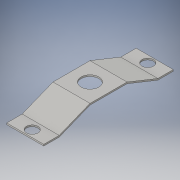
# Autodesk Inventor part: Up_cam_support
Saved by Autodesk Inventor 2016 (Build 200138000, 138)
## iProperties
Created: 2015-09-28
Part Number: Up_cam_support
Material: Generic
Document SubType Name: Modeling
Designer: fei
Density: 1 g/cm^3
Appearance: Default
Author: fei
Autodesk Inventor part; units mm, degrees
ref_plane "YZ Plane" through (0, 0, 0) normal (1, 0, 0) x (0, 1, 0)
ref_plane "XZ Plane" through (0, 0, 0) normal (0, 1, 0) x (-1, 0, 0)
ref_plane "XY Plane" through (0, 0, 0) normal (0, 0, 1) x (1, 0, 0)
sketch "Sketch1" plane through (0, 0, 0) normal (1, 0, 0) x (0, 1, 0)
  line L0 (174.9139, 1066.8) -> (200.3139, 1066.8)
  line L1 (200.3139, 1066.8) -> (200.3139, 812.8)
  line L2 (200.3139, 812.8) -> (403.5139, 304.8)
  line L3 (403.5139, 304.8) -> (403.5139, -304.8)
  line L4 (403.5139, -304.8) -> (200.3139, -812.8)
  line L5 (200.3139, -812.8) -> (200.3139, -1066.8)
  line L6 (174.9139, 1066.8) -> (174.9139, 812.8)
  line L7 (174.9139, 812.8) -> (378.1139, 304.8)
  line L8 (378.1139, 304.8) -> (378.1139, -304.8)
  line L9 (174.9139, -935.25) -> (174.9139, 993.0491) construction
  line L10 (174.9139, 681.698) -> (174.9139, -514.0179) construction
  line L11 (200.3139, -1066.8) -> (174.9139, -1066.8)
  line L12 (378.1139, -304.8) -> (174.9139, -812.8)
  line L13 (174.9139, -812.8) -> (174.9139, -1066.8)
  point P0 (0, 0)
  dimension "d0" = 254
  dimension "d1" = 508
  dimension "d2" = 609.6
  dimension "d3" = 508
  dimension "d4" = 254
  dimension "d6" = 304.8
  dimension "d8" = 25.4
  dimension "d10" = 203.2
  dimension "d26" = 25.4
  constraints: 28 end point, 6 point on line, 4 horizontal alignment, 3 vertical, 2 horizontal, 2 parallel, 1 collinear, 1 perpendicular
  measures "d0" distance of L0.end L1.end
  measures "d1" vertical distance of L1.end L2.end
  measures "d2" distance of L2.end L3.end
  measures "d3" vertical distance of L3.end L4.end
  measures "d4" distance of L4.end L5.end
  measures "d6" vertical distance of L2.end point (0, 0)
  measures "d8" distance of L0.start L0.end
  measures "d10" distance between parallel lines of L8 L9
  measures "d26" distance between parallel lines of L8 L3
extrude "Extrusion1" add sketch "Sketch1" along normal mid plane 609.6
sketch "Sketch2" plane through (-304.8, 200.3139, -812.8) normal (0, 1, 0) x (1, 0, 0)
  circle A0 centre (304.8, 139.7) radius 95.25
  line L0 (609.6, 254) -> (0, 254) projected
  line L1 (0, 0) -> (0, 254) projected
  circle A1 centre (304.8, -1765.3) radius 95.25
  line L2 (609.6, -1879.6) -> (0, -1879.6) projected
  line L3 (609.6, -1625.6) -> (609.6, -1879.6) projected
  point P0 (304.8, -812.8)
  dimension "d13" = 190.5
  dimension "d14" = 114.3
  dimension "d15" = 304.8
  dimension "d16" = 190.5
  dimension "d17" = 114.3
  dimension "d18" = 304.8
  constraints: 2 centre point
  measures "d13" diameter of A0
  measures "d14" distance from line of L0 A0.centre
  measures "d15" distance from line of L1 A0.centre
  measures "d16" diameter of A1
  measures "d17" distance from line of L2 A1.centre
  measures "d18" distance from line of L3 A1.centre
extrude "Extrusion2" cut sketch "Sketch2" against normal up to next
sketch "Sketch3" plane through (-304.8, 403.5139, 304.8) normal (0, 1, 0) x (1, 0, 0)
  circle A0 centre (304.8, 304.8) radius 146.05
  line L0 (0, 609.6) -> (0, 0) projected
  line L1 (609.6, 609.6) -> (0, 609.6) projected
  point P0 (304.8, 304.8)
  dimension "d21" = 292.1
  dimension "d22" = 304.8
  dimension "d23" = 304.8
  constraints: 1 centre point
  measures "d21" diameter of A0
  measures "d22" distance from line of L0 A0.centre
  measures "d23" distance from line of L1 A0.centre
extrude "Extrusion3" cut sketch "Sketch3" against normal up to next
body "Solid1"
